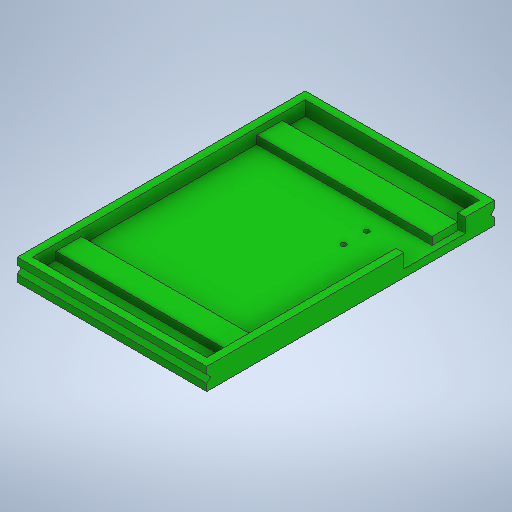
# Autodesk Inventor part: plate
Saved by Autodesk Inventor 2026.1 (Build 301233020, 233B)
## iProperties
Created: 2025-07-03
Part Number: plate
Material: Generic
Document SubType Name: Modeling
Designer: admin
Density: 1 g/cm^3
Appearance: Default
Author: admin
Autodesk Inventor part; units mm, degrees
ref_plane "YZ Plane" through (0, 0, 0) normal (1, 0, 0) x (0, 1, 0)
ref_plane "XZ Plane" through (0, 0, 0) normal (0, 1, 0) x (-1, 0, 0)
ref_plane "XY Plane" through (0, 0, 0) normal (0, 0, 1) x (1, 0, 0)
sketch "Sketch36" plane through (0, 0, 0) normal (0, 1, 0) x (-1, 0, 0)
  line L0 (29.1617, 36.148) -> (29.1617, -76.352)
  line L1 (29.1617, -76.352) -> (-44.8383, -76.352)
  line L2 (-44.8383, -76.352) -> (-44.8383, 36.148)
  line L3 (-44.8383, 36.148) -> (29.1617, 36.148)
  point P0 (0, 0)
  dimension "d191" = 112.5
  dimension "d192" = 74
  constraints: 8 end point, 3 perpendicular, 1 vertical
  measures "d191" distance of L0.start L0.end
  measures "d192" distance of L0.end L1.end
extrude "Extrusion21" add sketch "Sketch36" along normal blind 3
sketch "Sketch37" plane through (0, 3, 0) normal (0, 1, 0) x (1, 0, 0)
  line L0 (-29.1617, 76.352) -> (-29.1617, -36.148) projected
  line L1 (-29.1617, -36.148) -> (-29.1617, 76.352)
  line L2 (44.8383, -36.148) -> (44.8383, 76.352) projected
  line L3 (-29.1617, 76.352) -> (44.8383, 76.352)
  line L4 (44.8383, 76.352) -> (44.8383, -36.148)
  line L5 (-29.1617, -36.148) -> (44.8383, -36.148) projected
  line L6 (44.8383, -36.148) -> (-29.1617, -36.148)
  line L7 (-26.1617, -33.148) -> (41.8383, -33.148)
  line L8 (41.8383, 73.352) -> (-26.1617, 73.352)
  line L9 (-26.1617, 73.352) -> (-26.1617, -33.148)
  line L10 (41.8383, -33.148) -> (41.8383, 40.852)
  line L11 (41.8383, 40.852) -> (44.8383, 40.852)
  line L12 (41.8383, 73.352) -> (41.8383, 64.852)
  line L13 (41.8383, 64.852) -> (44.8383, 64.852)
  point P0 (0, 0)
  point P1 (43.3383, 64.852)
  dimension "d195" = 3
  dimension "d197" = 3
  dimension "d198" = 3
  dimension "d199" = 3
  dimension "d203" = 8.5
  dimension "d261" = 24
  constraints: 22 end point, 5 perpendicular, 3 point on line, 2 collinear, 1 horizontal, 1 midpoint, 1 parallel, 1 vertical
  measures "d195" distance between parallel lines of L9 L0
  measures "d197" distance between parallel lines of L3 L8
  measures "d198" distance between parallel lines of L7 L5
  measures "d199" distance between parallel lines of L2 L12
  measures "d203" distance of L8.start L12.end
  measures "d261" distance between parallel lines of L11 L13
extrude "Extrusion22" add sketch "Sketch37" along normal blind 5.5 contours L3 L2 L13 L12 L8 L9 L7 L10 L11 L5 L0
sketch "Sketch39" plane through (0, 0, 0) normal (0, -1, 0) x (1, 0, 0)
  circle A0 centre (8.3383, -20.852) radius 1.4 projected
  line L0 (-29.1617, -76.352) -> (-29.1617, 36.148) projected
  line L1 (44.8383, 36.148) -> (44.8383, -76.352) projected
  line L2 (-25.1617, -14.852) -> (-28.1617, -14.852)
  line L3 (-28.1617, -14.852) -> (-28.1617, -23.852)
  line L4 (-28.1617, -23.852) -> (-25.1617, -23.852)
  line L5 (-25.1617, -23.852) -> (-25.1617, -14.852)
  line L6 (-29.1617, 36.148) -> (44.8383, 36.148) projected
  point P0 (0, 0)
  dimension "d217" = 9
  dimension "d218" = 3
  dimension "d295" = 36.5
  dimension "d296" = 51
  constraints: 8 end point, 3 perpendicular, 1 horizontal
  measures "d217" distance of L4.end L2.start
  measures "d218" distance of L2.start L2.end
  measures "d295" distance from line of A0.centre L3
  measures "d296" distance between parallel lines of L6 L2
extrude "Extrusion25" add sketch "Sketch39" along normal blind 10 contours L5 L4 L3 L2
sketch "Sketch43" plane through (0, 0, 0) normal (0, -1, 0) x (1, 0, 0)
  circle A0 centre (24.8383, -37.352) radius 1
  circle A1 centre (24.8383, -46.352) radius 1
  line L0 (44.8383, -76.352) -> (-29.1617, -76.352) projected
  circle A2 centre (8.3383, -20.852) radius 1.4 projected
  line L1 (-29.1617, 36.148) -> (44.8383, 36.148) projected
  line L2 (44.8383, 36.148) -> (44.8383, -76.352) projected
  point P0 (0, 0)
  dimension "d252" = 2
  dimension "d253" = 2
  dimension "d254" = 9
  dimension "d256" = 30
  dimension "d258" = 20
  constraints: 2 centre point
  measures "d252" diameter of A0
  measures "d253" diameter of A1
  measures "d254" distance of A1.centre A0.centre
  measures "d256" distance from line of A1.centre L0
  measures "d258" distance from line of A1.centre L2
extrude "Extrusion29" cut sketch "Sketch43" against normal blind 10 contours A0 | A1
sketch "Sketch45" plane through (0, 3, 0) normal (0, 1, 0) x (1, 0, 0)
  line L0 (41.8383, -33.148) -> (41.8383, 40.852) projected
  line L1 (41.8383, -14.148) -> (-26.1617, -14.148)
  line L2 (-26.1617, 73.352) -> (-26.1617, -33.148) projected
  line L3 (-26.1617, -24.148) -> (41.8383, -24.148)
  line L4 (41.8383, -24.148) -> (41.8383, -14.148)
  line L5 (41.8383, -33.148) -> (-26.1617, -33.148) projected
  line L6 (-26.1617, 64.352) -> (42.4383, 64.352)
  line L7 (42.4383, 64.352) -> (42.4383, 54.352)
  line L8 (42.4383, 54.352) -> (-26.1617, 54.352)
  line L9 (-26.1617, 64.352) -> (-26.1617, 54.352)
  line L10 (-26.1617, 73.352) -> (41.8383, 73.352) projected
  point P0 (0, 0)
  point P1 (41.8383, -24.148)
  dimension "d274" = 10
  dimension "d275" = 9
  dimension "d276" = 9
  dimension "d277" = 10
  constraints: 14 end point, 5 point on line, 4 horizontal, 3 perpendicular
  measures "d274" distance between parallel lines of L3 L1
  measures "d275" distance between parallel lines of L3 L5
  measures "d276" distance between parallel lines of L10 L6
  measures "d277" distance between parallel lines of L6 L8
extrude "Extrusion31" add sketch "Sketch45" along normal blind 3 contours L2 L6 L7 L8 | L3 L2 L1 L0
sketch "Sketch48" plane through (-29.1617, 0, 36.148) normal (-1, 0, 0) x (0, 0, 1)
  circle A0 centre (-55.5, -5) radius 1.75
  line L0 (-51, 0) -> (-51, -10) projected
  line L1 (-51, -10) -> (-60, -10) projected
  point P0 (-36.148, 0)
  dimension "d297" = 3.5
  dimension "d298" = 4.5
  dimension "d299" = 5
  constraints: 1 centre point
  measures "d297" diameter of A0
  measures "d298" distance from line of A0.centre L0
  measures "d299" distance from line of L1 A0.centre
extrude "Extrusion34" cut sketch "Sketch48" against normal blind 10
sketch "Sketch50" plane through (44.8383, 0, 36.148) normal (1, 0, 0) x (0, 0, -1)
  line L0 (0, 0) -> (0, 8.5) projected
  line L1 (0, 5.75) -> (1.5, 4.25)
  line L2 (1.5, 4.25) -> (0, 2.75)
  line L3 (0, 8.5) -> (77, 8.5) projected
  point P0 (36.148, 0)
  dimension "d307" = 4.25
  dimension "d314" = 45
  dimension "d316" = 1.5
  constraints: 4 end point, 2 point on line, 1 perpendicular
  measures "d307" distance from line of L3 L1.end
  measures "d314" angle of L2 L0
  measures "d316" distance from line of L0 L1.end
extrude "Extrusion36" cut sketch "Sketch50" against normal blind 75
sketch "Sketch51" plane through (44.8383, 0, 36.148) normal (1, 0, 0) x (0, 0, -1)
  line L0 (112.5, 0) -> (112.5, 8.5) projected
  line L1 (112.5, 5.75) -> (111, 4.25)
  line L2 (111, 4.25) -> (112.5, 2.75)
  line L3 (101, 8.5) -> (112.5, 8.5) projected
  point P0 (36.148, 0)
  dimension "d317" = 45
  dimension "d318" = 45
  dimension "d319" = 4.25
  dimension "d320" = 1.5
  constraints: 4 end point, 2 point on line
  measures "d317" angle of L1 L0
  measures "d318" angle of L0 L2
  measures "d319" distance from line of L3 L1.end
  measures "d320" distance from line of L0 L1.end
extrude "Extrusion37" cut sketch "Sketch51" against normal blind 75
sketch "Sketch52" plane through (0, 0, 0) normal (0, -1, 0) x (1, 0, 0)
  circle A0 centre (8.3383, -20.852) radius 1.4 projected
  circle A1 centre (8.3383, -20.852) radius 1.4
  point P0 (0, 0)
  dimension "d324" = 2.8
  constraints: 1 centre point, 1 coincident
  measures "d324" diameter of A1
extrude "Extrusion38" add sketch "Sketch52" along normal blind 5
body "Solid2"
